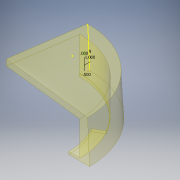
# Autodesk Inventor part: QuarterTop
Saved by Autodesk Inventor 2019 (Build 230136000, 136)
## iProperties
Created: 2019-10-06
Part Number: QuarterTop
Material: Generic
Document SubType Name: Modeling
Designer: james
Density: 1 g/cm^3
Appearance: Clear - Yellow
Author: james
Autodesk Inventor part; units mm, degrees
ref_plane "YZ Plane" through (0, 0, 0) normal (1, 0, 0) x (0, 1, 0)
ref_plane "XZ Plane" through (0, 0, 0) normal (0, 1, 0) x (-1, 0, 0)
ref_plane "XY Plane" through (0, 0, 0) normal (0, 0, 1) x (1, 0, 0)
sketch "Sketch1" plane through (0, 0, 0) normal (1, 0, 0) x (0, 1, 0)
  line L0 (74.9127, 161.4228) -> (59.7618, 161.4228)
  line L1 (-45.1093, -18.0862) -> (-45.1093, 9.0228)
  line L2 (-45.1093, 9.0228) -> (-51.4593, 9.0228)
  line L3 (-51.4593, 9.0228) -> (-51.4593, -41.7772)
  line L4 (37.2342, -18.0862) -> (-45.1093, -18.0862)
  line L5 (-51.4593, -41.7772) -> (50.0237, -36.9026)
  line L6 (50.0237, -36.9026) -> (74.9127, 161.4228)
  line L7 (59.7618, 161.4228) -> (37.2342, -18.0862)
  point P0 (0, 0)
  dimension "d0" = 101.6
  dimension "d2" = 50.8
  dimension "d3" = 6.35
  dimension "d4" = 87.25
  constraints: 16 end point, 2 perpendicular, 1 horizontal, 1 vertical
  measures "d0" distance of L3.end L5.end
  measures "d2" distance of L2.end L3.end
  measures "d3" distance between parallel lines of L3 L1
  measures "d4" angle of L3 L5
revolve "Revolution1" add sketch "Sketch1" angle 90 about axis through (0, 74.9127, 161.4228) along (0, -1, 0)
sketch "Sketch3" plane through (0, -51.4593, -41.7772) normal (0, -1, 0) x (1, 0, 0)
  arc A0 (0, 50.8) -> (152.4, 203.2) centre (0, 203.2) ccw projected
  arc A1 (0, 24.9755) -> (154.3469, 114.0878) centre (0, 203.2) ccw
  line L0 (198.3254, 203.2) -> (0, 203.2) projected
  arc A2 (0, 50.8) -> (131.9823, 127) centre (0, 203.2) ccw
  line L1 (0, 203.2) -> (0, 4.8746) projected
  line L2 (131.9823, 127) -> (154.3469, 114.0878)
  line L3 (0, 50.8) -> (0, 24.9755)
  point P0 (0, 41.7772)
  dimension "d11" = 30
  constraints: 6 point on circle, 4 end point, 2 centre point, 2 coincident, 1 point on line, 1 vertical
  measures "d11" angle of L0 L2
extrude "Extrusion2" cut sketch "Sketch3" against normal blind 25.4 contours A0 L2 A1 L1
sketch "Sketch4" plane through (0, -45.1093, -18.0862) normal (-1, 0, 0) x (0, 0, 1)
  line L0 (-18.8164, 95.133) -> (-23.6909, -6.35) projected
  point P0 (18.0862, 45.1093)
  point P1 (-10.1146, 11.5906)
  point P2 (-10.1146, 36.9906)
  dimension "d14" = 12.7
  dimension "d15" = 0
  dimension "d16" = 25.4
  measures "d14" distance from line of point (-10.115, 11.591) L0
  measures "d15" horizontal distance of point (-10.115, 11.591) point (-10.115, 36.991)
  measures "d16" distance of point (-10.115, 11.591) point (-10.115, 36.991)
body "Solid1"
